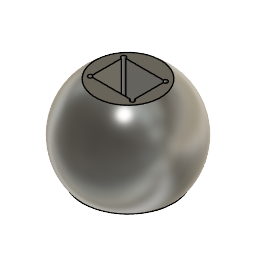
bead (Autodesk Fusion 360 design; units mm, degrees)
part number: 2025-11-02-13-53-45-732
Autodesk Fusion 360 part; units mm, degrees
note: some values were not read from the file. Set by a fixed rule: which sketch regions a step uses.
sketch "草图1" plane through (0, 0, 0) normal (0, 0, 1) x (1, 0, 0)
  circle A0 centre (0, 0) radius 1.985
  line L0 (-2, 0) -> (2, 0)
  dimension "d1" = 3.97
  constraint coincident A0.centre origin
  constraint horizontal L0
  measures "d1" diameter of A0
revolve "旋转1" add sketch "草图1" angle 360 about axis through (-2, 0, 0) along (1, 0, 0) contours A0 L0 picked at (0.4776, 0.5487)
sketch "草图2" plane through (0, 0, 0) normal (0, 0, 1) x (1, 0, 0)
  line L0 (0.7125, -0.5625) -> (-0.7125, -0.5625)
  line L1 (-0.7125, -0.5625) -> (-0.7125, 0.5625)
  line L2 (-0.7125, 0.5625) -> (0.7125, 0.5625)
  line L3 (0.7125, 0.5625) -> (0.7125, -0.5625)
  line L4 (0.7125, -0.5625) -> (-0.7125, 0.5625) construction
  line L5 (-0.7125, -0.5625) -> (0.7125, 0.5625) construction
  circle A0 centre (0.7125, -0.5625) radius 0.075
  circle A1 centre (0.7125, 0.5625) radius 0.075
  circle A2 centre (-0.7125, -0.5625) radius 0.075
  circle A3 centre (-0.7125, 0.5625) radius 0.075
  dimension "d3" = 1.425
  dimension "d4" = 1.125
  dimension "d12" = 0.15
  dimension "d13" = 0.15
  dimension "d14" = 0.15
  dimension "d15" = 0.15
  constraint horizontal L0
  constraint perpendicular L0 L1
  constraint parallel L0 L2
  constraint parallel L1 L3
  constraint coincident L4 origin
  constraint coincident L5 origin
  constraint coincident L0.start L3.end
  constraint coincident L2.end L3.start
  constraint coincident L0.end L1.start
  constraint coincident L1.end L2.start
  measures "d3" distance of L1.end L2.end
  measures "d4" distance of L0.end L1.end
  measures "d12" diameter of A0
  measures "d13" diameter of A1
  measures "d14" diameter of A2
  measures "d15" diameter of A3
extrude "拉伸1" cut sketch "草图2" along normal mid plane 3.8
sketch "草图3" plane through (0, 0, 0) normal (1, 0, 0) x (0, 1, 0)
  line L0 (-3.5, 3.5) -> (3.5, 3.5)
  line L1 (3.5, 3.5) -> (3.5, -3)
  line L2 (3.5, -3) -> (-3.5, -3)
  line L3 (-3.5, -3) -> (-3.5, 3.5)
  line L4 (-3.5, 0) -> (3.5, 0)
  line L5 (3.5, 0) -> (3.5, 1.65)
  line L6 (3.5, 1.65) -> (-3.5, 1.65)
  line L7 (-3.5, 1.65) -> (-3.5, 0)
  line L8 (-3.5, 0) -> (3.5, 0)
  line L9 (3.5, 0) -> (3.5, -1.25)
  line L10 (3.5, -1.25) -> (-3.5, -1.25)
  line L11 (-3.5, -1.25) -> (-3.5, 0)
  dimension "d20" = 1.65
  dimension "d21" = 1.25
  constraint horizontal L0
  constraint vertical L1
  constraint horizontal L2
  constraint vertical L3
  constraint horizontal L4
  constraint vertical L5
  constraint horizontal L6
  constraint vertical L7
  constraint coincident L3 L4.start
  constraint horizontal L8
  constraint vertical L9
  constraint horizontal L10
  constraint vertical L11
  measures "d20" distance of L4.start L6.end
  measures "d21" distance of L4.start L10.end
extrude "拉伸2" cut sketch "草图3" along normal mid plane 3.5 contours L0 L1 L3 L6 | L1 L2 L3 L10
